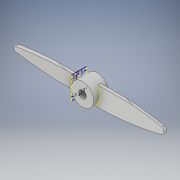
# Autodesk Inventor part: propeller
Saved by Autodesk Inventor 2018 (Build 220112000, 112)
## iProperties
Created: 2019-06-19
Part Number: propeller
Material: Generic
Document SubType Name: Modeling
Designer: Mike
Density: 1 g/cm^3
Appearance: Default
Author: Mike
Autodesk Inventor part; units mm, degrees
sketch "Sketch - Propeller Connecter" plane through (0, 0, 0) normal (0, 0, 1) x (1, 0, 0)
  circle A0 centre (0, 0) radius 7.5
  circle A1 centre (0, 0) radius 2.5
  dimension "d0" = 15
  dimension "d1" = 5
  constraints: 2 centre point, 2 coincident
  measures "d0" diameter of A0
  measures "d1" diameter of A1
extrude "Extrusion1" add sketch "Sketch - Propeller Connecter" along normal blind 10
ref_plane "Work Plane1" through (0, 7.5, 0) normal (0, 1, 0) x (-1, 0, 0)
ref_plane "Work Plane2" through (-7.5, 0, 0) normal (1, 0, 0) x (0, 1, 0)
sketch "Sketch3" plane through (-7.5, 0, 0) normal (1, 0, 0) x (0, 1, 0)
  line L0 (7.5, 10) -> (-7.5, 10) projected
  line L1 (7.5, 10) -> (7.5, 0)
  line L2 (7.5, 0) -> (7.5, 10) projected
  line L3 (-7.5, 0) -> (7.5, 0) projected
  line L4 (-7.5, 10) -> (-7.5, 0)
  line L5 (-7.5, 0) -> (-7.5, 10) projected
  line L6 (5.5, 7) -> (-5.5, 5)
  line L7 (5.5, 5) -> (-5.5, 3)
  line L8 (5.5, 5) -> (5.5, 7)
  line L9 (-5.5, 3) -> (-5.5, 5)
  point P0 (0, 0)
  point P1 (0, 5)
  dimension "d27" = 5
  dimension "d28" = 3
  dimension "d29" = 3
  dimension "d30" = 5
  dimension "d32" = 2
  dimension "d33" = 2
  dimension "d34" = 2
  dimension "d35" = 2
  constraints: 12 end point, 1 collinear, 1 point on line
  measures "d27" distance from line of L3 L7.start
  measures "d28" distance from line of L0 L6.start
  measures "d29" distance from line of L3 L7.end
  measures "d30" distance from line of L0 L6.end
  measures "d32" distance from line of L1 L6.start
  measures "d33" distance from line of L1 L7.start
  measures "d34" distance from line of L4 L6.end
  measures "d35" distance from line of L4 L7.end
sketch3d "3D Sketch2"
ref_plane "Work Plane3" through (7.5, 0, 0) normal (1, 0, 0) x (0, 1, 0)
sketch "Sketch4" plane through (7.5, 0, 0) normal (1, 0, 0) x (0, 1, 0)
  line L0 (5.5, 5) -> (-5.5, 7)
  line L1 (5.5, 3) -> (-5.5, 5)
  line L2 (5.5, 3) -> (5.5, 5)
  line L3 (-5.5, 5) -> (-5.5, 7)
  line L4 (7.5, 10) -> (-7.5, 10) projected
  line L5 (-7.5, 0) -> (7.5, 0) projected
  line L6 (-7.5, 0) -> (-7.5, 10)
  line L7 (7.5, 0) -> (7.5, 10)
  point P0 (0, 0)
  point P1 (0, 5)
  dimension "d38" = 3
  dimension "d39" = 5
  dimension "d40" = 3
  dimension "d42" = 5
  dimension "d43" = 2
  dimension "d44" = 2
  dimension "d45" = 2
  dimension "d46" = 2
  constraints: 12 end point, 2 vertical
  measures "d38" distance from line of L5 L1.start
  measures "d39" distance from line of L4 L0.start
  measures "d40" distance from line of L4 L0.end
  measures "d42" distance from line of L5 L1.end
  measures "d43" distance from line of L7 L1.start
  measures "d44" distance from line of L7 L0.start
  measures "d45" distance from line of L6 L1.end
  measures "d46" distance from line of L6 L0.end
sketch3d "3D Sketch3"
extrude "Extrusion2" add sketch "Sketch4" against normal blind 5 contours L2 L1 L3 L0
extrude "Extrusion3" add sketch "Sketch4" along normal blind 50 contours L2 L1 L3 L0
extrude "Extrusion4" add sketch "Sketch3" along normal blind 5 contours L8 L7 L9 L6
extrude "Extrusion5" add sketch "Sketch3" against normal blind 50 contours L8 L7 L9 L6
sketch "Sketch8" plane through (-5.099, -5.5, 3) normal (0, 0.1788854, -0.9838699) x (-1, 0, 0)
  line L0 (52.401, 0) -> (0, 0) projected
  line L1 (52.401, 11.1803) -> (52.401, 0) projected
  arc A0 (2.3083, 0) -> (52.401, 5.5902) centre (5.3498, 199.9769) ccw
  line L2 (52.401, 5.5902) -> (52.401, 0)
  line L3 (52.401, 0) -> (8.3914, 0)
  point P0 (-5.099, 4.8746)
  dimension "d59" = 200
  constraints: 4 end point, 3 point on circle, 2 point on line, 1 centre point, 1 collinear, 1 midpoint
  measures "d59" radius of A0
extrude "Extrusion6" cut sketch "Sketch8" against normal blind 30 contours L0 A0 L1
sketch "Sketch15" plane through (57.5, 5.5, 3) normal (0, -0.1788854, -0.9838699) x (-1, 0, 0)
  line L0 (52.401, -0.3578) -> (52.401, 0) projected
  arc A0 (52.401, 0) -> (-0.7421, -4.8746) centre (43.9347, -199.8207) ccw
  line L1 (-0.7421, -4.8746) -> (-0.7421, 0)
  line L2 (-0.7421, 0) -> (35.4685, 0)
  point P0 (57.5, -4.8746)
  dimension "d67" = 200
  constraints: 4 end point, 4 point on circle, 1 centre point, 1 perpendicular, 1 vertical
  measures "d67" radius of A0
extrude "Extrusion7" cut sketch "Sketch15" against normal blind 30
sketch "Sketch16" plane through (-57.5, 5.5, 7) normal (0, -0.1788854, 0.9838699) x (1, 0, 0)
  line L0 (52.401, -0.3578) -> (52.401, 0) projected
  line L1 (0, -5.9479) -> (0, 0) projected
  arc A0 (52.401, 0) -> (0, -5.9479) centre (48.5604, -199.9631) ccw
  line L2 (0, 0) -> (44.7198, 0)
  line L3 (52.401, 0) -> (0, 0) projected
  point P0 (57.5, -6.6635)
  dimension "d70" = 200
  constraints: 3 point on circle, 2 end point, 1 centre point, 1 point on line
  measures "d70" radius of A0
extrude "Extrusion8" cut sketch "Sketch16" against normal blind 30 contours L1 L2 A0
sketch "Sketch17" plane through (5.099, -5.5, 7) normal (0, 0.1788854, 0.9838699) x (1, 0, 0)
  ellipse E0 centre (-5.099, 5.5902) end of major axis (-5.099, -2.0328) minor radius 7.5 (0, 0) -> (0, 11.1803) ccw projected
  line L0 (52.401, 6.8321) -> (52.401, 0) projected
  arc A0 (0, 0) -> (52.401, 6.8321) centre (0.5699, 199.9992) ccw
  line L1 (52.401, 0) -> (1.1398, 0)
  line L2 (0, 0) -> (52.401, 0) projected
  point P0 (-5.099, 6.6635)
  dimension "d73" = 200
  constraints: 3 point on circle, 2 end point, 1 centre point, 1 point on line, 1 other
  measures "d73" radius of A0
extrude "Extrusion9" cut sketch "Sketch17" against normal blind 30
fillet "Fillet1" radius 2 1 edges at (57.5, 1.0459, 4.8098)
fillet "Fillet2" radius 2 1 edges at (-57.5, -0.176, 4.968)
body "Solid1"
